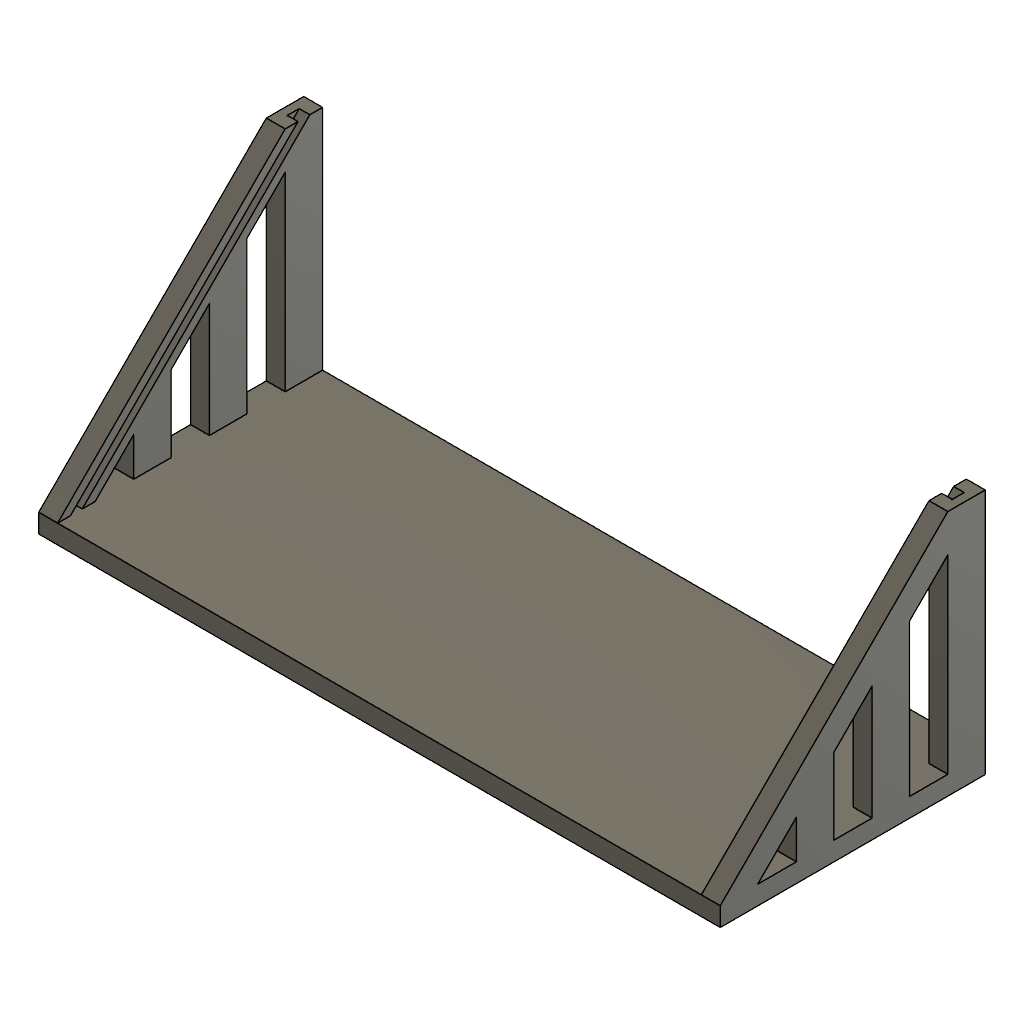
MirrorSupport (Autodesk Fusion 360 design; units mm, degrees)
Autodesk Fusion 360 part; units mm, degrees
sketch "Sketch1" plane through (0, 0, 0) normal (0, 1, 0) x (1, 0, 0)
  line L0 (0, 0) -> (180, 0)
  line L1 (180, 0) -> (180, 70)
  line L2 (180, 70) -> (0, 70)
  line L3 (0, 70) -> (0, 0)
  dimension "d1" = 180
  dimension "d2" = 70
  constraint horizontal L0
  constraint vertical L1
  constraint horizontal L2
  constraint vertical L3
  constraint coincident L0.start L3.end
  measures "d1" distance of L0.start L0.end
  measures "d2" distance of L0.start L2.end
extrude "Extrude1" add sketch "Sketch1" along normal blind 5
sketch "Sketch2" plane through (0, 0, 0) normal (-1, 0, 0) x (0, 0, 1)
  line L0 (-70, 0) -> (0, 0)
  line L1 (0, 0) -> (0, 5)
  line L2 (0, 5) -> (-70, 5)
  line L3 (-70, 5) -> (-70, 0)
  line L4 (-70, 5) -> (-70, 105) construction
  line L5 (0, 5) -> (-70, 75)
  line L6 (-9.8995, 5) -> (-70, 65.1005)
  line L7 (-70, 65.1005) -> (-60.1005, 65.1005)
  line L8 (-9.8995, 5) -> (0, 5)
  dimension "d5" = 100
  dimension "d6" = 45
  constraint coincident L2.end L3.start
  constraint perpendicular L2 L4
  constraint coincident L1.end L2.start
  constraint coincident L4 L5.end
  constraint coincident L2 L6.start
  constraint coincident L4 L6.end
  constraint coincident L5 L7.end
  constraint perpendicular L4 L7
  measures "d5" distance of L2.end L4.end
  measures "d6" angle of L2 L5
extrude "Extrude2" add sketch "Sketch2" against normal blind 5 contours L2 L5 L6 L7 L8
ref_plane "WorkPlane1" through (2.5, 65.1005, -70) normal (0, -0.707107, 0.707107) x (1, 0, 0)
sketch "Sketch3" plane through (0, 67.5503, -67.5503) normal (0, -0.707107, 0.707107) x (1, 0, 0)
  line L0 (0, -3.4645) -> (0, 3.5355) construction
  line L1 (0, 3.5355) -> (5, 3.5355) construction
  line L2 (5, 3.5355) -> (5, -3.4645) construction
  line L3 (5, -3.4645) -> (0, -3.4645) construction
  line L4 (5, 1.1355) -> (2.2, 1.1355)
  line L5 (2.2, 1.1355) -> (2.2, -1.0645)
  line L6 (2.2, -1.0645) -> (5, -1.0645)
  line L7 (5, -1.0645) -> (5, 1.1355)
  line L8 (5, 0.0355) -> (5, 3.5355)
  line L9 (5, 0.0355) -> (5, -3.4645)
  dimension "d11" = 2.8
  dimension "d12" = 2.2
  constraint horizontal L4
  constraint vertical L5
  constraint horizontal L6
  constraint vertical L7
  constraint coincident L2 L4.start
  constraint midpoint L7 L8.start
  constraint coincident L1.end L2.start
  constraint coincident L2.end L3.start
  constraint equal L8 L9
  measures "d11" distance of L4.start L4.end
  measures "d12" distance of L4.start L6.end
extrude "Extrude3" cut sketch "Sketch3" along normal up to surface end surface through (0, 5, 0) normal (0, 1, 0) offset 0
sketch "Sketch4" plane through (0, 5, 0) normal (0, 1, 0) x (-1, 0, 0)
  line L0 (0, -9.8995) -> (-5, -9.8995)
  line L1 (-5, -9.8995) -> (-5, -6.5054)
  line L2 (-5, -6.5054) -> (-2.2, -6.5054)
  line L3 (-2.2, -6.5054) -> (-2.2, -3.3941)
  line L4 (-2.2, -3.3941) -> (-5, -3.3941)
  line L5 (-5, -3.3941) -> (-5, 0)
  line L6 (-5, 0) -> (-180, 0)
  line L7 (-180, 0) -> (-180, -70)
  line L8 (-180, -70) -> (0, -70)
  line L9 (0, -70) -> (0, -9.8995)
  line L10 (-2.2, -66.6059) -> (-5, -66.6059)
  line L11 (-5, -66.6059) -> (-5, -70)
  line L12 (-5, -70) -> (0, -70)
  line L13 (0, -70) -> (0, -60.1005)
  line L14 (0, -60.1005) -> (-5, -60.1005)
  line L15 (-5, -60.1005) -> (-5, -63.4946)
  line L16 (-5, -63.4946) -> (-2.2, -63.4946)
  line L17 (-2.2, -63.4946) -> (-2.2, -66.6059)
  line L18 (-5, -66.6059) -> (-2.2, -66.6059)
  line L19 (-2.2, -66.6059) -> (-2.2, -6.5054)
  line L20 (-2.2, -6.5054) -> (-5, -6.5054)
  line L21 (-5, -6.5054) -> (-5, -66.6059)
  line L22 (-5, -60.1005) -> (0, -60.1005)
  line L23 (0, -60.1005) -> (0, -70)
  line L24 (0, -70) -> (-5, -70)
  line L25 (-5, -70) -> (-5, -60.1005)
  line L26 (-5, -40.1005) -> (0, -40.1005)
  line L27 (-5, -50) -> (-5, -40.1005)
  line L28 (0, -40.1005) -> (0, -50)
  line L29 (0, -50) -> (-5, -50)
  line L30 (-5, -20.1005) -> (0, -20.1005)
  line L31 (-5, -30) -> (-5, -20.1005)
  line L32 (0, -20.1005) -> (0, -30)
  line L33 (0, -30) -> (-5, -30)
  dimension "d19" = 20
  dimension "d20" = 0
  constraint horizontal L22
  constraint vertical L23
  constraint horizontal L24
  constraint vertical L25
  constraint coincident L8.end L9.start
  constraint coincident L14.end L15.start
extrude "Extrude4" add sketch "Sketch4" along normal up to surface contours L9 L19 L30 L32 L33 | L19 L21 L30 L31 L33 | L9 L19 L26 L28 L29 | L19 L21 L26 L27 L29 | L8 L9 L10 L11 L12 L13 L14 L17 L18 L19 L22 L23 L24 L25 | L14 L15 L16 L19 L21 L22 L25 | L10 L16 L17 L18 L19 L21 L25 end surface through (0, 5, -9.8995) normal (0, -0.707107, -0.707107) offset 0
ref_plane "WorkPlane2" through (90, 32.5503, -35) normal (-1, 0, 0) x (0, 0, 1)
mirror "Mirror1" about plane through (90, 32.5503, -35) normal (-1, 0, 0) of "Extrude2", "Extrude3", "Extrude4"
sketch "Sketch5" plane through (0, 0, 0) normal (0, -1, 0) x (1, 0, 0)
  line L0 (0, 0) -> (0, -70)
  line L1 (0, -70) -> (180, -70)
  line L2 (180, -70) -> (180, 0)
  line L3 (180, 0) -> (0, 0)
  line L4 (180, -35) -> (0, -35) construction
  line L5 (90, -70) -> (90, 0) construction
  circle A0 centre (140, -35) radius 15.5
  circle A1 centre (40, -35) radius 15.5
  dimension "d23" = 31
  dimension "d24" = 50
  constraint midpoint L2 L4.start
  constraint midpoint L0 L4.end
  constraint midpoint L1 L5.start
  constraint midpoint L3 L5.end
  constraint coincident L4 A0.centre
  constraint symmetric L5 A0 A1
  measures "d23" diameter of A0
  measures "d24" distance of L5 A0.centre
extrude "Extrude5" cut sketch "Sketch5" against normal blind 2.5 contours A0 | A1
